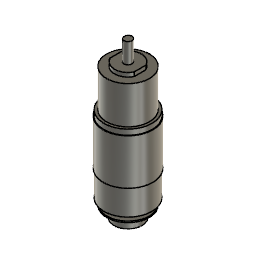
Moteur (Autodesk Fusion 360 design; units mm, degrees)
Autodesk Fusion 360 part; units mm, degrees
sketch "Sketch1" plane through (0, 0, 0) normal (0, 0, 1) x (1, 0, 0)
  circle A0 centre (0, 0) radius 10.5
  dimension "d1" = 21
  constraint coincident A0.centre origin
  measures "d1" diameter of A0
extrude "Extrude1" add sketch "Sketch1" along normal blind 5
sketch "Sketch2" plane through (0, 0, 5) normal (0, 0, 1) x (-1, 0, 0)
  circle A0 centre (0, 0) radius 10.5
  circle A1 centre (0, 0) radius 4
  dimension "d4" = 8
  constraint coincident A0.centre A1.centre
  measures "d4" diameter of A1
extrude "Extrude2" add sketch "Sketch2" along normal blind 3 contours A1
sketch "Sketch3" plane through (0, 0, 8) normal (0, 0, 1) x (-1, 0, 0)
  circle A0 centre (0, 0) radius 4
  circle A1 centre (0, 0) radius 16
  dimension "d7" = 32
  constraint coincident A0.centre A1.centre
  measures "d7" diameter of A1
extrude "Extrude3" add sketch "Sketch3" along normal blind 1 contours A0 | A1
sketch "Sketch4" plane through (0, 0, 9) normal (0, 0, 1) x (-1, 0, 0)
  circle A0 centre (0, 0) radius 16
  circle A1 centre (0, 0) radius 7.5
  dimension "d10" = 15
  constraint coincident A0.centre A1.centre
  measures "d10" diameter of A1
extrude "Extrude4" add sketch "Sketch4" along normal blind 4 contours A1
sketch "Sketch5" plane through (0, 0, 13) normal (0, 0, 1) x (-1, 0, 0)
  circle A0 centre (0, 0) radius 7.5
  circle A1 centre (0, 0) radius 18
  dimension "d13" = 36
  constraint coincident A0.centre A1.centre
  measures "d13" diameter of A1
extrude "Extrude5" add sketch "Sketch5" along normal blind 19 contours A0 | A1
sketch "Sketch6" plane through (0, 0, 32) normal (0, 0, 1) x (-1, 0, 0)
  circle A0 centre (0, 0) radius 18
  circle A1 centre (0, 0) radius 18.5
  dimension "d16" = 37
  constraint coincident A0.centre A1.centre
  measures "d16" diameter of A1
extrude "Extrude6" add sketch "Sketch6" along normal blind 34 contours A0 | A1
sketch "Sketch7" plane through (0, 0, 66) normal (0, 0, 1) x (-1, 0, 0)
  circle A0 centre (0, 0) radius 18.5
  circle A1 centre (0, 0) radius 18
  dimension "d19" = 36
  constraint coincident A0.centre A1.centre
  measures "d19" diameter of A1
extrude "Extrude7" add sketch "Sketch7" along normal blind 4 contours A1
sketch "Sketch8" plane through (0, 0, 70) normal (0, 0, 1) x (-1, 0, 0)
  circle A0 centre (0, 0) radius 18
  circle A1 centre (0, 0) radius 16
  dimension "d22" = 32
  constraint coincident A0.centre A1.centre
  measures "d22" diameter of A1
extrude "Extrude8" add sketch "Sketch8" along normal blind 28 contours A1
sketch "Sketch9" plane through (0, 0, 98) normal (0, 0, 1) x (-1, 0, 0)
  circle A0 centre (0, 0) radius 16
  line L0 (0, -10) -> (0, 10) construction
  line L1 (9, -4.3589) -> (9, 4.3589)
  line L2 (-9, -4.3589) -> (-9, 4.3589)
  arc A1 (9, 4.3589) -> (-9, 4.3589) centre (0, 0) ccw
  arc A2 (-9, -4.3589) -> (9, -4.3589) centre (0, 0) ccw
  dimension "d25" = 20
  dimension "d26" = 9
  constraint coincident A0.centre A1.centre
  constraint coincident L0.start A1
  constraint coincident L0.end A1
  constraint vertical L0
  constraint vertical L1
  constraint symmetric L0 L1.start L2.start
  constraint symmetric L0 L1.end L2.end
  constraint concentric A1 A2
  measures "d25" diameter of A1
  measures "d26" distance of L0 L1
sketch "Sketch10" plane through (0, 0, 98) normal (0, 0, 1) x (-1, 0, 0)
extrude "Extrude9" add sketch "Sketch9" along normal blind 3 contours L1 L2 A1 A2
sketch "Sketch11" plane through (0, 0, 101) normal (0, 0, 1) x (-1, 0, 0)
  arc A0 (-9, -4.3589) -> (9, -4.3589) centre (0, 0) ccw
  line L0 (9, -4.3589) -> (9, 4.3589)
  arc A1 (9, 4.3589) -> (-9, 4.3589) centre (0, 0) ccw
  line L1 (-9, 4.3589) -> (-9, -4.3589)
  circle A2 centre (0, 0) radius 3
  dimension "d29" = 6
  constraint coincident A0.centre A1.centre
  measures "d29" diameter of A2
extrude "Extrude10" add sketch "Sketch11" along normal blind 4 contours A2
sketch "Sketch12" plane through (0, 0, 105) normal (0, 0, 1) x (-1, 0, 0)
  circle A0 centre (0, 0) radius 3
  line L0 (2.7017, -1.3042) -> (2.7017, 1.3042)
  arc A1 (2.7017, 1.3042) -> (2.7017, -1.3042) centre (0, 0) ccw
  constraint coincident A0.centre A1.centre
  constraint vertical L0
extrude "Extrude11" add sketch "Sketch12" along normal blind 11 contours A0 L0 A1
